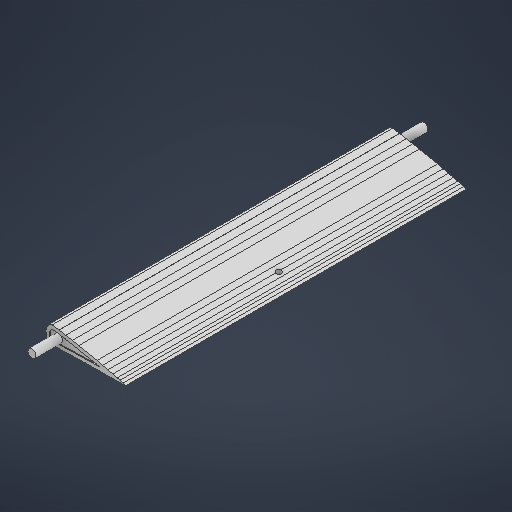
# Autodesk Inventor part: Aileronn
Saved by Autodesk Inventor 2026 (Build 300175050, 175E)
## iProperties
Created: 2026-02-20
Part Number: Aileronn
Material: Všeobecné
Document SubType Name: Modeling
Designer: marti
Density: 1 g/cm^3
Appearance: Výchozí
Author: marti
Autodesk Inventor part; units mm, degrees
ref_plane "YZ Plane" through (0, 0, 0) normal (1, 0, 0) x (0, 1, 0)
sketch "Náčrt1" plane through (0, 0, 0) normal (0, 0, 1) x (1, 0, 0)
  line L0 (0, 0.000851) -> (0.094911, -0.580945)
  line L1 (0.094911, -0.580945) -> (0.396989, -1.143314)
  line L2 (0.396989, -1.143314) -> (0.894048, -1.645981)
  line L3 (0.894048, -1.645981) -> (1.581057, -2.09068)
  line L4 (1.581057, -2.09068) -> (2.453483, -2.479327)
  line L5 (2.453483, -2.479327) -> (3.506939, -2.813773)
  line L6 (3.506939, -2.813773) -> (4.73698, -3.095871)
  line L7 (4.73698, -3.095871) -> (6.139089, -3.327507)
  line L8 (6.139089, -3.327507) -> (7.708609, -3.510745)
  line L9 (7.708609, -3.510745) -> (9.440802, -3.647809)
  line L10 (9.440802, -3.647809) -> (11.330785, -3.741093)
  line L11 (11.330785, -3.741093) -> (13.373713, -3.793261)
  line L12 (13.373713, -3.793261) -> (15.564024, -3.793261)
  line L13 (15.564024, -3.793261) -> (17.897264, -3.793261)
  line L14 (17.897264, -3.793261) -> (20.367571, -3.741017)
  line L15 (20.367571, -3.741017) -> (22.971162, -3.685954)
  line L16 (22.971162, -3.685954) -> (25.69841, -3.553961)
  line L17 (25.69841, -3.553961) -> (28.546484, -3.41612)
  line L18 (28.546484, -3.41612) -> (29.828031, -3.354095)
  line L19 (29.828031, -3.354095) -> (25.26931, -3.575379)
  line L20 (25.26931, -3.575379) -> (37.753063, -2.962959)
  line L21 (37.753063, -2.962959) -> (41.025913, -2.800972)
  line L22 (41.025913, -2.800972) -> (44.853912, -2.611508)
  line L23 (44.853912, -2.611508) -> (35.101831, -3.022599)
  line L24 (35.101831, -3.022599) -> (60.437501, -1.969901)
  line L25 (60.437501, -1.969901) -> (54.928831, -2.193826)
  line L26 (54.928831, -2.193826) -> (58.573799, -2.045517)
  line L27 (58.573799, -2.045517) -> (62.271081, -1.89508)
  line L28 (62.271081, -1.89508) -> (73.029725, -1.457291)
  line L29 (73.029725, -1.457291) -> (71.483231, -1.521548)
  line L30 (71.483231, -1.521548) -> (73.599961, -1.434996)
  line L31 (73.599961, -1.434996) -> (77.422315, -1.282568)
  line L32 (77.422315, -1.282568) -> (84.76267, -1.001041)
  line L33 (87.29246, -0.912541) -> (102.918601, -0.349582)
  line L34 (102.918601, -0.349582) -> (98.182211, -0.524007)
  line L35 (98.182211, -0.524007) -> (96.406676, -0.57204)
  line L36 (96.406676, -0.57204) -> (100.096747, -0.480208)
  line L37 (100.096747, -0.480208) -> (103.712753, -0.394718)
  line L38 (103.712753, -0.394718) -> (107.248074, -0.313312)
  line L39 (107.248074, -0.313312) -> (110.674764, -0.240584)
  line L40 (110.674764, -0.240584) -> (113.957246, -0.170916)
  line L41 (113.957246, -0.170916) -> (117.106646, -0.202793)
  line L42 (117.106646, -0.202793) -> (120.063576, -0.165865)
  line L43 (120.063576, -0.165865) -> (122.79977, -0.136027)
  line L44 (122.79977, -0.136027) -> (127.200216, -0.093877)
  line L45 (127.200216, -0.093877) -> (127.395492, -0.097122)
  line L46 (127.395492, -0.097122) -> (129.073471, -0.125007)
  line L47 (129.073471, -0.125007) -> (129.997389, -0.14036)
  line L48 (129.997389, -0.14036) -> (129.999721, 0)
  line L49 (129.999721, 0) -> (128.618258, 0.589205)
  line L50 (128.618258, 0.589205) -> (126.804845, 1.039503)
  line L51 (126.804845, 1.039503) -> (125.261376, 1.445959)
  line L52 (125.261376, 1.445959) -> (122.79551, 2.078606)
  line L53 (122.79551, 2.078606) -> (120.059849, 2.759791)
  line L54 (120.059849, 2.759791) -> (117.102842, 3.471969)
  line L55 (117.102842, 3.471969) -> (113.977352, 4.266244)
  line L56 (113.977352, 4.266244) -> (110.66531, 4.930661)
  line L57 (110.66531, 4.930661) -> (107.23303, 5.619197)
  line L58 (107.23303, 5.619197) -> (103.702173, 6.327509)
  line L59 (103.702173, 6.327509) -> (100.086993, 7.051724)
  line L60 (100.086993, 7.051724) -> (96.430757, 7.706157)
  line L61 (96.430757, 7.706157) -> (92.657875, 8.383215)
  line L62 (92.657875, 8.383215) -> (87.912368, 9.13793)
  line L63 (82.48975, 9.99733) -> (81.248528, 10.173239)
  line L64 (81.248528, 10.173239) -> (77.419756, 10.673011)
  line L65 (77.419756, 10.673011) -> (73.597963, 11.127907)
  line L66 (73.597963, 11.127907) -> (69.793227, 11.53573)
  line L67 (69.793227, 11.53573) -> (66.015076, 11.894556)
  line L68 (66.015076, 11.894556) -> (62.272544, 12.202786)
  line L69 (62.272544, 12.202786) -> (58.574303, 12.459094)
  line L70 (58.574303, 12.459094) -> (54.928585, 12.662453)
  line L71 (54.928585, 12.662453) -> (51.343326, 12.811654)
  line L72 (51.343326, 12.811654) -> (47.826137, 12.889004)
  line L73 (47.826137, 12.889004) -> (44.384348, 12.886924)
  line L74 (44.384348, 12.886924) -> (41.025005, 12.807468)
  line L75 (41.025005, 12.807468) -> (37.754972, 12.653158)
  line L76 (37.754972, 12.653158) -> (34.580853, 12.426945)
  line L77 (34.580853, 12.426945) -> (31.509044, 12.1323)
  line L78 (31.509044, 12.1323) -> (28.545785, 11.773045)
  line L79 (28.545785, 11.773045) -> (25.697134, 11.353444)
  line L80 (25.697134, 11.353444) -> (22.968954, 10.878112)
  line L81 (22.968954, 10.878112) -> (20.367004, 10.351976)
  line L82 (20.367004, 10.351976) -> (17.896861, 9.780249)
  line L83 (17.896861, 9.780249) -> (15.563985, 9.168391)
  line L84 (15.563985, 9.168391) -> (13.373719, 8.521992)
  line L85 (13.373719, 8.521992) -> (11.331263, 7.846772)
  line L86 (11.331263, 7.846772) -> (9.441726, 7.148529)
  line L87 (9.441726, 7.148529) -> (7.710087, 6.43297)
  line L88 (7.710087, 6.43297) -> (6.14126, 5.70575)
  line L89 (6.14126, 5.70575) -> (4.740029, 4.972303)
  line L90 (4.740029, 4.972303) -> (3.511113, 4.237816)
  line L91 (3.511113, 4.237816) -> (2.459114, 3.507112)
  line L92 (2.459114, 3.507112) -> (1.588582, 2.784585)
  line L93 (1.588582, 2.784585) -> (0.903976, 2.074122)
  line L94 (0.903976, 2.074122) -> (0.409677, 1.378986)
  line L95 (0.409677, 1.378986) -> (0.111307, 0.704744)
  line L96 (0.111307, 0.704744) -> (0, 0.000851)
  line L97 (41.095797, 10.808583) -> (44.408602, 10.886939)
  line L98 (44.408602, 10.886939) -> (47.804752, 10.888991)
  line L99 (47.804752, 10.888991) -> (51.279754, 10.812569)
  line L100 (51.279754, 10.812569) -> (54.831307, 10.66477)
  line L101 (54.831307, 10.66477) -> (58.449464, 10.462949)
  line L102 (58.449464, 10.462949) -> (62.121317, 10.20847)
  line L103 (62.121317, 10.20847) -> (65.83844, 9.902332)
  line L104 (65.83844, 9.902332) -> (69.592094, 9.545833)
  line L105 (69.592094, 9.545833) -> (73.373185, 9.140544)
  line L106 (73.373185, 9.140544) -> (77.172123, 8.688369)
  line L107 (77.172123, 8.688369) -> (80.978767, 8.191485)
  line L108 (80.978767, 8.191485) -> (82.122439, 8.029401)
  line L109 (92.324146, 6.411152) -> (96.077934, 5.737521)
  line L110 (96.077934, 5.737521) -> (99.714338, 5.086637)
  line L111 (99.714338, 5.086637) -> (103.309061, 4.36652)
  line L112 (103.309061, 4.36652) -> (106.823521, 3.661498)
  line L113 (106.823521, 3.661498) -> (110.23815, 2.976502)
  line L114 (110.23815, 2.976502) -> (113.534078, 2.315319)
  line L115 (113.534078, 2.315319) -> (115.5088, 1.813486)
  line L116 (115.5088, 1.813486) -> (113.946145, 1.829302)
  line L117 (113.946145, 1.829302) -> (110.632325, 1.75897)
  line L118 (110.632325, 1.75897) -> (107.203835, 1.686203)
  line L119 (107.203835, 1.686203) -> (103.666097, 1.604742)
  line L120 (103.666097, 1.604742) -> (100.048232, 1.519208)
  line L121 (100.048232, 1.519208) -> (96.354754, 1.42729)
  line L122 (96.354754, 1.42729) -> (98.118365, 1.475001)
  line L123 (98.118365, 1.475001) -> (102.864558, 1.649787)
  line L124 (102.864558, 1.649787) -> (88.185356, 1.120939)
  line L125 (81.687483, 0.882487) -> (77.344743, 0.715928)
  line L126 (77.344743, 0.715928) -> (73.519259, 0.563376)
  line L127 (73.519259, 0.563376) -> (71.400862, 0.476755)
  line L128 (71.400862, 0.476755) -> (72.947553, 0.54102)
  line L129 (72.947553, 0.54102) -> (62.189768, 0.103267)
  line L130 (62.189768, 0.103267) -> (58.49249, -0.04717)
  line L131 (58.49249, -0.04717) -> (54.84756, -0.195477)
  line L132 (54.84756, -0.195477) -> (60.355371, 0.028412)
  line L133 (60.355371, 0.028412) -> (35.0182, -1.024348)
  line L134 (35.0182, -1.024348) -> (44.76236, -0.613592)
  line L135 (44.76236, -0.613592) -> (40.926284, -0.803455)
  line L136 (40.926284, -0.803455) -> (37.654631, -0.965383)
  line L137 (37.654631, -0.965383) -> (25.171828, -1.577756)
  line L138 (25.171828, -1.577756) -> (29.731206, -1.35644)
  line L139 (29.731206, -1.35644) -> (28.456303, -1.418143)
  line L140 (28.456303, -1.418143) -> (25.608229, -1.555984)
  line L141 (25.608229, -1.555984) -> (22.901664, -1.686977)
  line L142 (22.901664, -1.686977) -> (20.318778, -1.741602)
  line L143 (20.318778, -1.741602) -> (17.876117, -1.793261)
  line L144 (17.876117, -1.793261) -> (15.564024, -1.793261)
  line L145 (15.564024, -1.793261) -> (13.399245, -1.793261)
  line L146 (13.399245, -1.793261) -> (11.40562, -1.742352)
  line L147 (11.40562, -1.742352) -> (9.569008, -1.651702)
  line L148 (9.569008, -1.651702) -> (7.903518, -1.519916)
  line L149 (7.903518, -1.519916) -> (6.418202, -1.346509)
  line L150 (6.418202, -1.346509) -> (5.123881, -1.13268)
  line L151 (5.123881, -1.13268) -> (4.033953, -0.882715)
  line L152 (4.033953, -0.882715) -> (3.165219, -0.606914)
  line L153 (3.165219, -0.606914) -> (2.537136, -0.327117)
  line L154 (2.537136, -0.327117) -> (2.163323, -0.085149)
  line L155 (2.163323, -0.085149) -> (2.032217, 0.047436)
  line L156 (2.032217, 0.047436) -> (2.045955, 0.134309)
  line L157 (2.045955, 0.134309) -> (2.15678, 0.384746)
  line L158 (2.15678, 0.384746) -> (2.447553, 0.793663)
  line L159 (2.447553, 0.793663) -> (2.95154, 1.316685)
  line L160 (2.95154, 1.316685) -> (3.670472, 1.913387)
  line L161 (3.670472, 1.913387) -> (4.59588, 2.556162)
  line L162 (4.59588, 2.556162) -> (5.717577, 3.226568)
  line L163 (5.717577, 3.226568) -> (7.026074, 3.911475)
  line L164 (7.026074, 3.911475) -> (8.512907, 4.600687)
  line L165 (8.512907, 4.600687) -> (10.170515, 5.285654)
  line L166 (10.170515, 5.285654) -> (11.991969, 5.958739)
  line L167 (11.991969, 5.958739) -> (13.970814, 6.612929)
  line L168 (13.970814, 6.612929) -> (16.10086, 7.241556)
  line L169 (16.10086, 7.241556) -> (18.376152, 7.838311)
  line L170 (18.376152, 7.838311) -> (20.790778, 8.397188)
  line L171 (20.790778, 8.397188) -> (23.338863, 8.912433)
  line L172 (23.338863, 8.912433) -> (26.014559, 9.37862)
  line L173 (26.014559, 9.37862) -> (28.81191, 9.790665)
  line L174 (28.81191, 9.790665) -> (31.724914, 10.143827)
  line L175 (31.724914, 10.143827) -> (34.747447, 10.433745)
  line L176 (34.747447, 10.433745) -> (37.873214, 10.656513)
  line L177 (37.873214, 10.656513) -> (41.095797, 10.808583)
  line L178 (0, 16.225457) -> (0, -7.129714)
  line L179 (-109.521987, 0) -> (169.920006, 0)
  arc A0 (85.411458, 9.53532) -> (84.76267, -1.001041) centre (91.861806, 3.849977) ccw
  arc A1 (87.920288, 9.143837) -> (87.29246, -0.912541) centre (91.861806, 3.849977) ccw
  line L180 (85.411458, 9.53532) -> (82.48975, 9.99733)
  arc A2 (92.702807, 8.375152) -> (92.612792, 8.390385) centre (91.890292, 3.84744) ccw
  line L181 (88.551007, 7.011224) -> (92.324146, 6.411152)
  arc A3 (82.122439, 8.029401) -> (81.687483, 0.882487) centre (91.861806, 3.849977) ccw
  arc A4 (88.551007, 7.011224) -> (88.185356, 1.120939) centre (91.890292, 3.84744) ccw
  point P0 (0, 0)
  point P1 (0.00916, 0.044316)
  point P2 (80.023721, 10.392523)
  point P3 (81.248526, -1.146055)
  point P4 (85.078349, -0.99229)
  point P5 (0, -1.830216)
  point P6 (0, -1.831382)
  point P7 (72.218592, -1.489825)
  point P8 (-4.203174, 0)
  point P9 (0, 0.170199)
  point P10 (129.761686, -0.162984)
  point P11 (0, 11.007127)
  point P12 (0, -1.829889)
  point P13 (41.358731, -2.74491)
  point P14 (41.276972, -0.746582)
  point P15 (0, 8.995671)
  point P16 (0, 0.171754)
  point P17 (0, 0.171447)
  point P18 (-69.601702, 0)
  point P19 (72.137779, 0.508541)
  point P20 (26.158294, -1.529362)
  point P21 (59.651791, 0)
  point P22 (2.079124, 0)
  point P23 (26.255634, -3.526992)
  point P24 (44.112323, -2.648213)
  point P25 (44.021374, -0.650266)
  point P26 (59.656423, 0)
  point P27 (97.434787, 1.454169)
  point P28 (97.496892, -0.544909)
  point P29 (97.760074, -0.535427)
  point P30 (87.912368, 9.13793)
  point P31 (97.695504, 1.463561)
  point P32 (59.671573, 0)
  dimension "d0" = 2
  dimension "d1" = 0
  dimension "d10" = 129.99972
  dimension "d12" = 3.84744
  dimension "d13" = 91.89029
  dimension "d17" = 6.60004
  constraints: 360 end point, 12 collinear, 11 point on circle, 5 centre point, 3 coincident, 3 point on line, 2 parallel, 2 perpendicular, 2 tangent, 1 horizontal, 75 other
  measures "d0" distance between parallel lines of L74 L97
  measures "d1" distance from line of L178 point (0, 0.001)
  measures "d10" distance of L48.end point (0, 0.001)
  measures "d12" distance from line of L179 A2.centre
  measures "d13" distance from line of L178 A2.centre
  measures "d17" radius of A1
ref_plane "Pracovní rovina1" through (0, 0, 50) normal (0, 0, 1) x (1, 0, 0)
sketch "Náčrt2" plane through (0.119749, -0.0139, 50) normal (0, 0, 1) x (1, 0, 0)
  line L0 (-71.730261, -0.320975) -> (-71.63535, -0.901921)
  line L1 (-71.63535, -0.901921) -> (-71.333272, -1.464289)
  line L2 (-71.333272, -1.464289) -> (-70.836213, -1.966957)
  line L3 (-70.836213, -1.966957) -> (-70.149204, -2.411656)
  line L4 (-70.149204, -2.411656) -> (-69.276778, -2.800303)
  line L5 (-69.276778, -2.800303) -> (-68.223322, -3.134748)
  line L6 (-68.223322, -3.134748) -> (-66.993281, -3.416846)
  line L7 (-66.993281, -3.416846) -> (-65.591173, -3.648482)
  line L8 (-65.591173, -3.648482) -> (-64.021652, -3.83172)
  line L9 (-64.021652, -3.83172) -> (-62.289459, -3.968784)
  line L10 (-62.289459, -3.968784) -> (-60.399477, -4.062068)
  line L11 (-60.399477, -4.062068) -> (-58.356548, -4.114236)
  line L12 (-58.356548, -4.114236) -> (-56.166238, -4.114236)
  line L13 (-56.166238, -4.114236) -> (-53.832998, -4.114236)
  line L14 (-53.832998, -4.114236) -> (-51.36269, -4.061992)
  line L15 (-51.36269, -4.061992) -> (-48.75917, -4.006931)
  line L16 (-48.75917, -4.006931) -> (-46.031852, -3.874935)
  line L17 (-46.031852, -3.874935) -> (-43.183777, -3.737094)
  line L18 (-43.183777, -3.737094) -> (-40.217881, -3.59355)
  line L19 (-40.217881, -3.59355) -> (-37.150015, -3.4367)
  line L20 (-37.150015, -3.4367) -> (-33.974542, -3.27718)
  line L21 (-33.974542, -3.27718) -> (-30.704925, -3.110406)
  line L22 (-30.704925, -3.110406) -> (-27.34602, -2.939077)
  line L23 (-27.34602, -2.939077) -> (-23.905442, -2.795356)
  line L24 (-23.905442, -2.795356) -> (-23.405529, -2.775231)
  line L25 (-23.405529, -2.775231) -> (-16.802017, -2.514825)
  line L26 (-16.802017, -2.514825) -> (-13.156462, -2.366492)
  line L27 (-13.156462, -2.366492) -> (-9.458981, -2.216047)
  line L28 (-9.458981, -2.216047) -> (1.299588, -1.776116)
  line L29 (1.299588, -1.776116) -> (-1.938992, -1.906491)
  line L30 (-1.938992, -1.906491) -> (1.867532, -1.756977)
  line L31 (1.867532, -1.756977) -> (5.691255, -1.606787)
  line L32 (5.691255, -1.606787) -> (13.346033, -1.320295)
  line L33 (13.346033, -1.320295) -> (17.155494, -1.188385)
  line L34 (17.155494, -1.188385) -> (20.937886, -1.067637)
  line L35 (20.937886, -1.067637) -> (24.680381, -0.957075)
  line L36 (24.680381, -0.957075) -> (28.368562, -0.857229)
  line L37 (28.368562, -0.857229) -> (31.986169, -0.76835)
  line L38 (31.986169, -0.76835) -> (35.516622, -0.69035)
  line L39 (35.516622, -0.69035) -> (38.940495, -0.622915)
  line L40 (38.940495, -0.622915) -> (42.233802, -0.565546)
  line L41 (42.233802, -0.565546) -> (45.376334, -0.568497)
  line L42 (45.376334, -0.568497) -> (48.333873, -0.531564)
  line L43 (48.333873, -0.531564) -> (51.069996, -0.501729)
  line L44 (51.069996, -0.501729) -> (53.536291, -0.478108)
  line L45 (53.536291, -0.478108) -> (55.664534, -0.460038)
  line L46 (55.664534, -0.460038) -> (57.342964, -0.445787)
  line L47 (57.342964, -0.445787) -> (58.27195, -0.4379)
  line L48 (58.27195, -0.4379) -> (58.26946, -0.144571)
  line L49 (58.26946, -0.144571) -> (57.336498, 0.110873)
  line L50 (57.336498, 0.110873) -> (55.658373, 0.562338)
  line L51 (55.658373, 0.562338) -> (53.530524, 1.122684)
  line L52 (53.530524, 1.122684) -> (51.064675, 1.755326)
  line L53 (51.064675, 1.755326) -> (48.329032, 2.436507)
  line L54 (48.329032, 2.436507) -> (45.371995, 3.148692)
  line L55 (45.371995, 3.148692) -> (42.248339, 3.946544)
  line L56 (42.248339, 3.946544) -> (38.935199, 4.610431)
  line L57 (38.935199, 4.610431) -> (35.502769, 5.298222)
  line L58 (35.502769, 5.298222) -> (31.970784, 6.005961)
  line L59 (31.970784, 6.005961) -> (28.356016, 6.727176)
  line L60 (28.356016, 6.727176) -> (24.666501, 7.390521)
  line L61 (24.666501, 7.390521) -> (20.927539, 8.061822)
  line L62 (20.927539, 8.061822) -> (17.143303, 8.663326)
  line L63 (17.143303, 8.663326) -> (10.759488, 9.676355)
  line L64 (10.759488, 9.676355) -> (9.518266, 9.852264)
  line L65 (9.518266, 9.852264) -> (5.689495, 10.352036)
  line L66 (5.689495, 10.352036) -> (1.867702, 10.806932)
  line L67 (1.867702, 10.806932) -> (-1.937034, 11.214755)
  line L68 (-1.937034, 11.214755) -> (-5.715185, 11.573581)
  line L69 (-5.715185, 11.573581) -> (-9.457717, 11.881811)
  line L70 (-9.457717, 11.881811) -> (-13.155958, 12.138119)
  line L71 (-13.155958, 12.138119) -> (-16.801676, 12.341478)
  line L72 (-16.801676, 12.341478) -> (-20.386935, 12.490679)
  line L73 (-20.386935, 12.490679) -> (-23.904124, 12.568029)
  line L74 (-23.904124, 12.568029) -> (-27.345913, 12.565949)
  line L75 (-27.345913, 12.565949) -> (-30.705256, 12.486493)
  line L76 (-30.705256, 12.486493) -> (-33.975289, 12.332183)
  line L77 (-33.975289, 12.332183) -> (-37.149408, 12.10597)
  line L78 (-37.149408, 12.10597) -> (-40.221217, 11.811325)
  line L79 (-40.221217, 11.811325) -> (-43.184476, 11.45207)
  line L80 (-43.184476, 11.45207) -> (-46.033127, 11.032469)
  line L81 (-46.033127, 11.032469) -> (-48.761307, 10.557137)
  line L82 (-48.761307, 10.557137) -> (-51.363257, 10.031001)
  line L83 (-51.363257, 10.031001) -> (-53.8334, 9.459274)
  line L84 (-53.8334, 9.459274) -> (-56.166276, 8.847416)
  line L85 (-56.166276, 8.847416) -> (-58.356542, 8.201017)
  line L86 (-58.356542, 8.201017) -> (-60.398998, 7.525797)
  line L87 (-60.398998, 7.525797) -> (-62.288535, 6.827554)
  line L88 (-62.288535, 6.827554) -> (-64.020174, 6.111995)
  line L89 (-64.020174, 6.111995) -> (-65.589001, 5.384775)
  line L90 (-65.589001, 5.384775) -> (-66.990232, 4.651328)
  line L91 (-66.990232, 4.651328) -> (-68.219148, 3.916841)
  line L92 (-68.219148, 3.916841) -> (-69.271147, 3.186137)
  line L93 (-69.271147, 3.186137) -> (-70.141679, 2.46361)
  line L94 (-70.141679, 2.46361) -> (-70.826285, 1.753147)
  line L95 (-70.826285, 1.753147) -> (-71.320584, 1.058011)
  line L96 (-71.320584, 1.058011) -> (-71.618133, 0.385625)
  line L97 (-71.618133, 0.385625) -> (-71.730261, -0.320975)
  line L98 (-30.634464, 10.487608) -> (-27.32166, 10.565963)
  line L99 (-27.32166, 10.565963) -> (-23.925509, 10.568016)
  line L100 (-23.925509, 10.568016) -> (-20.450507, 10.491593)
  line L101 (-20.450507, 10.491593) -> (-16.898954, 10.343795)
  line L102 (-16.898954, 10.343795) -> (-13.280797, 10.141973)
  line L103 (-13.280797, 10.141973) -> (-9.608944, 9.887494)
  line L104 (-9.608944, 9.887494) -> (-5.891822, 9.581357)
  line L105 (-5.891822, 9.581357) -> (-2.138168, 9.224857)
  line L106 (-2.138168, 9.224857) -> (1.642923, 8.819569)
  line L107 (1.642923, 8.819569) -> (5.441862, 8.367393)
  line L108 (5.441862, 8.367393) -> (9.248505, 7.87051)
  line L109 (9.248505, 7.87051) -> (10.462422, 7.69847)
  line L110 (10.462422, 7.69847) -> (16.829598, 6.688082)
  line L111 (16.829598, 6.688082) -> (20.59381, 6.089761)
  line L112 (20.59381, 6.089761) -> (24.312829, 5.42204)
  line L113 (24.312829, 5.42204) -> (27.983365, 4.762107)
  line L114 (27.983365, 4.762107) -> (31.578647, 4.04478)
  line L115 (31.578647, 4.04478) -> (35.09326, 3.340522)
  line L116 (35.09326, 3.340522) -> (38.508038, 2.656269)
  line L117 (38.508038, 2.656269) -> (41.804083, 1.995807)
  line L118 (41.804083, 1.995807) -> (44.008348, 1.432788)
  line L119 (44.008348, 1.432788) -> (42.217323, 1.43447)
  line L120 (42.217323, 1.43447) -> (38.903386, 1.376742)
  line L121 (38.903386, 1.376742) -> (35.474842, 1.309215)
  line L122 (35.474842, 1.309215) -> (31.93952, 1.231108)
  line L123 (31.93952, 1.231108) -> (28.316939, 1.142106)
  line L124 (28.316939, 1.142106) -> (24.62379, 1.042125)
  line L125 (24.62379, 1.042125) -> (20.876449, 0.931421)
  line L126 (20.876449, 0.931421) -> (17.08898, 0.810511)
  line L127 (17.08898, 0.810511) -> (13.274026, 0.678411)
  line L128 (13.274026, 0.678411) -> (5.614607, 0.391744)
  line L129 (5.614607, 0.391744) -> (1.789036, 0.241482)
  line L130 (1.789036, 0.241482) -> (-2.018464, 0.091929)
  line L131 (-2.018464, 0.091929) -> (1.218507, 0.22224)
  line L132 (1.218507, 0.22224) -> (-9.540493, -0.217709)
  line L133 (-9.540493, -0.217709) -> (-13.237772, -0.368146)
  line L134 (-13.237772, -0.368146) -> (-16.882076, -0.516428)
  line L135 (-16.882076, -0.516428) -> (-23.485157, -0.776817)
  line L136 (-23.485157, -0.776817) -> (-23.987402, -0.797036)
  line L137 (-23.987402, -0.797036) -> (-27.438699, -0.941205)
  line L138 (-27.438699, -0.941205) -> (-30.804555, -1.112888)
  line L139 (-30.804555, -1.112888) -> (-34.075655, -1.279738)
  line L140 (-34.075655, -1.279738) -> (-37.251247, -1.439263)
  line L141 (-37.251247, -1.439263) -> (-40.317283, -1.59602)
  line L142 (-40.317283, -1.59602) -> (-43.273959, -1.739117)
  line L143 (-43.273959, -1.739117) -> (-46.122033, -1.876958)
  line L144 (-46.122033, -1.876958) -> (-48.828668, -2.007954)
  line L145 (-48.828668, -2.007954) -> (-51.411484, -2.062577)
  line L146 (-51.411484, -2.062577) -> (-53.854144, -2.114236)
  line L147 (-53.854144, -2.114236) -> (-56.166238, -2.114236)
  line L148 (-56.166238, -2.114236) -> (-58.331017, -2.114236)
  line L149 (-58.331017, -2.114236) -> (-60.324642, -2.063327)
  line L150 (-60.324642, -2.063327) -> (-62.161253, -1.972677)
  line L151 (-62.161253, -1.972677) -> (-63.826744, -1.840891)
  line L152 (-63.826744, -1.840891) -> (-65.312059, -1.667484)
  line L153 (-65.312059, -1.667484) -> (-66.60638, -1.453655)
  line L154 (-66.60638, -1.453655) -> (-67.696309, -1.203691)
  line L155 (-67.696309, -1.203691) -> (-68.565043, -0.92789)
  line L156 (-68.565043, -0.92789) -> (-69.193125, -0.648093)
  line L157 (-69.193125, -0.648093) -> (-69.566938, -0.406125)
  line L158 (-69.566938, -0.406125) -> (-69.697755, -0.273831)
  line L159 (-69.697755, -0.273831) -> (-69.683709, -0.185314)
  line L160 (-69.683709, -0.185314) -> (-69.573482, 0.063771)
  line L161 (-69.573482, 0.063771) -> (-69.282708, 0.472688)
  line L162 (-69.282708, 0.472688) -> (-68.778721, 0.99571)
  line L163 (-68.778721, 0.99571) -> (-68.059789, 1.592411)
  line L164 (-68.059789, 1.592411) -> (-67.134381, 2.235187)
  line L165 (-67.134381, 2.235187) -> (-66.012684, 2.905592)
  line L166 (-66.012684, 2.905592) -> (-64.704187, 3.590499)
  line L167 (-64.704187, 3.590499) -> (-63.217355, 4.279712)
  line L168 (-63.217355, 4.279712) -> (-61.559747, 4.964679)
  line L169 (-61.559747, 4.964679) -> (-59.738293, 5.637763)
  line L170 (-59.738293, 5.637763) -> (-57.759448, 6.291954)
  line L171 (-57.759448, 6.291954) -> (-55.629402, 6.92058)
  line L172 (-55.629402, 6.92058) -> (-53.354109, 7.517336)
  line L173 (-53.354109, 7.517336) -> (-50.939484, 8.076213)
  line L174 (-50.939484, 8.076213) -> (-48.391398, 8.591457)
  line L175 (-48.391398, 8.591457) -> (-45.715702, 9.057645)
  line L176 (-45.715702, 9.057645) -> (-42.918352, 9.469689)
  line L177 (-42.918352, 9.469689) -> (-40.005347, 9.822852)
  line L178 (-40.005347, 9.822852) -> (-36.982815, 10.11277)
  line L179 (-36.982815, 10.11277) -> (-33.857048, 10.335537)
  line L180 (-33.857048, 10.335537) -> (-30.634464, 10.487608)
  line L181 (0, 15.904482) -> (0, -7.450689)
  line L182 (-97.730704, 0) -> (84.272393, 0)
  point P0 (0, 0)
  point P1 (-71.721101, -0.27666)
  point P2 (9.518265, -1.467031)
  point P3 (0, -1.829258)
  point P4 (0, -1.830331)
  point P5 (-0.665209, -1.856459)
  point P6 (-4.216396, 0)
  point P7 (0, 0.171211)
  dimension "d6" = 2
  dimension "d5" = 71.73026
  constraints: 366 end point, 12 collinear, 3 perpendicular, 2 parallel, 1 coincident, 1 horizontal, 82 other
  measures "d6" distance between parallel lines of L75 L98
  measures "d5" distance from line of L181 point (-71.73, -0.321)
extrude "Vysunutí2" [suppressed]
ref_plane "Pracovní rovina3" through (0, 0, 0) normal (0, 0, 1) x (1, 0, 0)
sketch "Náčrt1 outline for Vysunutí8" plane through (0, 0, 0) normal (0, 0, 1) x (1, 0, 0)
  line L0 (103.702173, 6.327509) -> (100.086993, 7.051724)
  line L1 (107.23303, 5.619197) -> (103.702173, 6.327509)
  line L2 (110.66531, 4.930661) -> (107.23303, 5.619197)
  line L3 (113.977352, 4.266244) -> (110.66531, 4.930661)
  line L4 (117.102842, 3.471969) -> (113.977352, 4.266244)
  line L5 (120.059849, 2.759791) -> (117.102842, 3.471969)
  line L6 (122.79551, 2.078606) -> (120.059849, 2.759791)
  line L7 (125.261376, 1.445959) -> (122.79551, 2.078606)
  line L8 (126.804845, 1.039503) -> (125.261376, 1.445959)
  line L9 (128.618258, 0.589205) -> (126.804845, 1.039503)
  line L10 (129.999721, 0) -> (128.618258, 0.589205)
  line L11 (129.997389, -0.14036) -> (129.999721, 0)
  line L12 (129.073471, -0.125007) -> (129.997389, -0.14036)
  line L13 (127.395492, -0.097122) -> (129.073471, -0.125007)
  line L14 (127.200216, -0.093877) -> (127.395492, -0.097122)
  line L15 (122.79977, -0.136027) -> (127.200216, -0.093877)
  line L16 (120.063576, -0.165865) -> (122.79977, -0.136027)
  line L17 (117.106646, -0.202793) -> (120.063576, -0.165865)
  line L18 (113.957246, -0.170916) -> (117.106646, -0.202793)
  line L19 (110.674764, -0.240584) -> (113.957246, -0.170916)
  line L20 (107.248074, -0.313312) -> (110.674764, -0.240584)
  line L21 (103.712753, -0.394718) -> (107.248074, -0.313312)
  line L22 (100.096747, -0.480208) -> (103.712753, -0.394718)
  line L23 (97.496892, -0.544909) -> (100.096747, -0.480208)
  line L24 (87.29246, -0.912541) -> (97.496892, -0.544909)
  arc A0 (87.912368, 9.13793) -> (87.29246, -0.912541) centre (91.861806, 3.849977) ccw
  line L25 (92.612792, 8.390385) -> (87.912368, 9.13793)
  arc A1 (92.702807, 8.375152) -> (92.612792, 8.390385) centre (91.890292, 3.84744) ccw
  line L26 (96.430757, 7.706157) -> (92.702807, 8.375152)
  line L27 (100.086993, 7.051724) -> (96.430757, 7.706157)
  line L28 (97.760074, -0.535427) -> (97.496892, -0.544909)
  line L29 (96.406676, -0.57204) -> (97.760074, -0.535427)
  line L30 (97.496892, -0.544909) -> (96.406676, -0.57204)
  line L31 (98.182211, -0.524007) -> (97.760074, -0.535427)
  line L32 (102.918601, -0.349582) -> (98.182211, -0.524007)
  line L33 (97.760074, -0.535427) -> (102.918601, -0.349582)
  line L34 (103.666097, 1.604742) -> (100.048232, 1.519208)
  line L35 (107.203835, 1.686203) -> (103.666097, 1.604742)
  line L36 (110.632325, 1.75897) -> (107.203835, 1.686203)
  line L37 (113.946145, 1.829302) -> (110.632325, 1.75897)
  line L38 (115.5088, 1.813486) -> (113.946145, 1.829302)
  line L39 (113.534078, 2.315319) -> (115.5088, 1.813486)
  line L40 (110.23815, 2.976502) -> (113.534078, 2.315319)
  line L41 (106.823521, 3.661498) -> (110.23815, 2.976502)
  line L42 (103.309061, 4.36652) -> (106.823521, 3.661498)
  line L43 (99.714338, 5.086637) -> (103.309061, 4.36652)
  line L44 (96.077934, 5.737521) -> (99.714338, 5.086637)
  line L45 (92.324146, 6.411152) -> (96.077934, 5.737521)
  line L46 (88.551007, 7.011224) -> (92.324146, 6.411152)
  arc A2 (88.185356, 1.120939) -> (88.551007, 7.011224) centre (91.890292, 3.84744) cw
  line L47 (97.434787, 1.454169) -> (88.185356, 1.120939)
  line L48 (100.048232, 1.519208) -> (97.434787, 1.454169)
extrude "Vysunutí8" add sketch "Náčrt1 outline for Vysunutí8" along normal mid plane 191
fillet "Zaoblení7" radius 2 4 edges at (88.551, 7.0112, 0) (88.1854, 1.1209, 0) (87.2925, -0.9125, 0) (87.9124, 9.1379, 0)
sketch "Náčrt4" plane through (0, 0, 0) normal (0, 0, 1) x (1, 0, 0)
  arc A0 (88.838293, 8.990673) -> (87.073029, 8.391797) centre (88.524165, 7.015496) ccw
  arc A1 (87.073029, 8.391797) -> (86.549727, -0.06695) centre (91.861806, 3.849977) ccw
  arc A2 (86.549727, -0.06695) -> (88.231445, -0.878713) centre (88.159439, 1.119991) ccw
  line L0 (88.231445, -0.878713) -> (97.496892, -0.544909)
  line L1 (97.496892, -0.544909) -> (96.406676, -0.57204)
  line L2 (96.406676, -0.57204) -> (97.760074, -0.535427)
  line L3 (97.760074, -0.535427) -> (102.918601, -0.349582)
  line L4 (102.918601, -0.349582) -> (98.182211, -0.524007)
  line L5 (98.182211, -0.524007) -> (97.760074, -0.535427)
  line L6 (97.760074, -0.535427) -> (97.496892, -0.544909)
  line L7 (97.496892, -0.544909) -> (100.096747, -0.480208)
  line L8 (100.096747, -0.480208) -> (103.712753, -0.394718)
  line L9 (103.712753, -0.394718) -> (107.248074, -0.313312)
  line L10 (107.248074, -0.313312) -> (113.957246, -0.170916)
  line L11 (113.957246, -0.170916) -> (117.106646, -0.202793)
  line L12 (117.106646, -0.202793) -> (120.063576, -0.165865)
  line L13 (120.063576, -0.165865) -> (122.79977, -0.136027)
  line L14 (122.79977, -0.136027) -> (127.200216, -0.093877)
  line L15 (127.200216, -0.093877) -> (129.997389, -0.14036)
  line L16 (129.997389, -0.14036) -> (129.999721, 0)
  line L17 (129.999721, 0) -> (128.618258, 0.589205)
  line L18 (128.618258, 0.589205) -> (126.804845, 1.039503)
  line L19 (126.804845, 1.039503) -> (125.261376, 1.445959)
  line L20 (125.261376, 1.445959) -> (122.79551, 2.078606)
  line L21 (122.79551, 2.078606) -> (120.059849, 2.759791)
  line L22 (120.059849, 2.759791) -> (117.102842, 3.471969)
  line L23 (117.102842, 3.471969) -> (113.977352, 4.266244)
  line L24 (113.977352, 4.266244) -> (103.702173, 6.327509)
  line L25 (103.702173, 6.327509) -> (100.086993, 7.051724)
  line L26 (100.086993, 7.051724) -> (96.430757, 7.706157)
  line L27 (96.430757, 7.706157) -> (92.702807, 8.375152)
  arc A3 (92.702807, 8.375152) -> (92.612792, 8.390385) centre (91.890292, 3.84744) ccw
  line L28 (92.612792, 8.390385) -> (88.838293, 8.990673)
  line L29 (103.666097, 1.604742) -> (100.048232, 1.519208)
  line L30 (100.048232, 1.519208) -> (97.434787, 1.454169)
  line L31 (97.434787, 1.454169) -> (89.453332, 1.16662)
  arc A4 (87.451378, 2.640627) -> (89.453332, 1.16662) centre (89.381324, 3.165324) ccw
  arc A5 (87.636717, 5.598854) -> (87.451378, 2.640627) centre (91.890292, 3.84744) ccw
  arc A6 (89.80021, 6.812553) -> (87.636717, 5.598854) centre (89.486082, 4.837376) ccw
  line L32 (89.80021, 6.812553) -> (92.324146, 6.411152)
  line L33 (92.324146, 6.411152) -> (96.077934, 5.737521)
  line L34 (96.077934, 5.737521) -> (99.714338, 5.086637)
  line L35 (99.714338, 5.086637) -> (103.309061, 4.36652)
  line L36 (103.309061, 4.36652) -> (113.534078, 2.315319)
  line L37 (113.534078, 2.315319) -> (115.5088, 1.813486)
  line L38 (115.5088, 1.813486) -> (113.946145, 1.829302)
  line L39 (113.946145, 1.829302) -> (107.203835, 1.686203)
  line L40 (107.203835, 1.686203) -> (103.666097, 1.604742)
  line L41 (96.077934, 5.737521) -> (92.324146, 6.411152)
  circle A7 centre (91.890292, 3.84744) radius 2.25
  point P0 (0, 0)
  dimension "d61" = 4.5
  constraints: 1 centre point, 1 coincident
  measures "d61" diameter of A7
extrude "Vysunutí10" add sketch "Náčrt4" along normal mid plane 220 contours A7
extrude "Vysunutí11" add sketch "Náčrt4" along normal mid plane 190 contours L29 L30 L31 A4 A5 A6 L32 L33 L34 L35 L36 L37 L38 L39 L40 | A7
sketch "Náčrt5" plane through (117.102842, 3.471969, 95.5) normal (0.234149, 0.9722007, 0) x (0.9722007, -0.234149, 0)
  circle A0 centre (3.351314, 95.5) radius 1.5
  line L0 (-3.224582, 0) -> (-13.696761, 0)
  line L1 (-13.696761, 191) -> (-3.224582, 191)
  line L2 (13.351314, 191) -> (13.351314, 0)
  point P0 (-113.03451, 95.5)
  dimension "d62" = 3
  dimension "d63" = 95.5
  dimension "d64" = 191
  dimension "d65" = 10
  constraints: 1 centre point
  measures "d62" diameter of A0
  measures "d63" distance from line of L0 A0.centre
  measures "d64" distance between parallel lines of L1 L0
  measures "d65" distance from line of L2 A0.centre
extrude "Vysunutí12" cut sketch "Náčrt5" against normal through all
